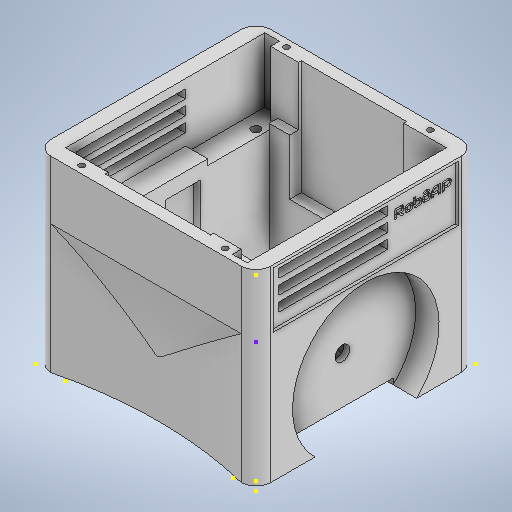
# Autodesk Inventor part: Chassi_VSSS
Saved by Autodesk Inventor 2025.2 (Build 292293000, 293)
## iProperties
Created: 2025-03-20
Part Number: Chassi_VSSS
Material: Genérico
Document SubType Name: Modeling
Designer: miche
Density: 1 g/cm^3
Appearance: Padrão
Author: miche
Autodesk Inventor part; units mm, degrees
(part 1 of 2)
ref_plane "YZ Plane" through (0, 0, 0) normal (1, 0, 0) x (0, 1, 0)
ref_plane "XZ Plane" through (0, 0, 0) normal (0, 1, 0) x (-1, 0, 0)
ref_plane "XY Plane" through (0, 0, 0) normal (0, 0, 1) x (1, 0, 0)
sketch "Esboço1" plane through (0, 0, 0) normal (0, 1, 0) x (-1, 0, 0)
  line L0 (5, 0) -> (70, 0)
  line L1 (75, -5) -> (75, -70)
  line L2 (70, -75) -> (5, -75)
  line L3 (0, -70) -> (0, -5)
  arc A0 (75, -5) -> (70, 0) centre (70, -5) ccw
  arc A1 (70, -75) -> (75, -70) centre (70, -70) ccw
  arc A2 (0, -70) -> (5, -75) centre (5, -70) ccw
  arc A3 (5, 0) -> (0, -5) centre (5, -5) ccw
  point P0 (0, 0)
  point P1 (75, -75)
  point P2 (75, 0)
  point P3 (0, -75)
  dimension "d0" = 75
  dimension "d1" = 75
  dimension "d2" = 5
  dimension "d3" = 5
  constraints: 8 end point, 8 point on circle, 8 point on line, 8 tangent, 4 centre point, 2 equal radius, 2 parallel, 1 horizontal, 1 perpendicular
  measures "d0" distance of point (75, -75) point (0, -75)
  measures "d1" distance of point (75, 0) point (75, -75)
  measures "d2" radius of A0
  measures "d3" radius of A3
extrude "Extrusão1" add sketch "Esboço1" along normal blind 3
sketch "Esboço2" plane through (0, 3, 0) normal (0, 1, 0) x (1, 0, 0)
  arc A0 (-70, 75) -> (-75, 70) centre (-70, 70) ccw projected
  line L0 (-70, 75) -> (-70, 70)
  line L1 (-70, 70) -> (-75, 70)
  line L2 (-70, 70) -> (-70, 5)
  line L3 (-70, 5) -> (-75, 5)
  line L4 (-75, 5) -> (-75, 70)
  line L5 (-70, 70) -> (-5, 70)
  line L6 (-5, 70) -> (-5, 5)
  line L7 (-5, 5) -> (-70, 5)
  line L8 (-5, 70) -> (0, 70)
  line L9 (0, 70) -> (0, 5)
  line L10 (0, 5) -> (-5, 5)
  line L11 (-5, 5) -> (-5, 0)
  line L12 (-5, 0) -> (-70, 0)
  line L13 (-70, 0) -> (-70, 5)
  line L14 (-5, 75) -> (-70, 75) projected
  line L15 (-5, 75) -> (-5, 70)
  arc A1 (-70, 75) -> (-75, 70) centre (-70, 70) ccw
  arc A2 (0, 70) -> (-5, 75) centre (-5, 70) ccw projected
  arc A3 (0, 70) -> (-5, 75) centre (-5, 70) ccw
  arc A4 (-5, 0) -> (0, 5) centre (-5, 5) ccw projected
  arc A5 (-5, 0) -> (0, 5) centre (-5, 5) ccw
  arc A6 (-75, 5) -> (-70, 0) centre (-70, 5) ccw
  line L16 (-70, 70) -> (-65, 70)
  line L17 (-65, 70) -> (-65, 5)
  line L18 (-65, 5) -> (-70, 5)
  line L19 (-70, 5) -> (-70, 70)
  line L20 (-5, 70) -> (-10, 70)
  line L21 (-10, 70) -> (-10, 5)
  line L22 (-10, 5) -> (-5, 5)
  line L23 (-5, 5) -> (-5, 70)
  line L24 (-70, 70) -> (-70, 71)
  line L25 (-70, 70) -> (-5, 70)
  line L26 (-5, 70) -> (-5, 71)
  line L27 (-5, 71) -> (-70, 71)
  line L28 (-70, 71) -> (-70, 70)
  line L29 (-70, 5) -> (-5, 5)
  line L30 (-5, 5) -> (-5, 4)
  line L31 (-5, 4) -> (-70, 4)
  line L32 (-70, 4) -> (-70, 5)
  arc A7 (-70, 75) -> (-5, 75) centre (-37.5, 205.0313) ccw
  arc A8 (-5, 0) -> (-70, 0) centre (-37.5, -130.0312) ccw
  point P0 (0, 0)
  constraints: 64 end point, 13 perpendicular, 13 point on circle, 10 point on line, 9 parallel, 6 centre point, 5 horizontal, 2 tangent, 2 vertical
extrude "Extrusão2" add sketch "Esboço2" along normal blind 15 contours L1 L2 L3 L4 | L5 L17 L7 L2 | L9 L10 L6 L8 | L6 L7 L21 L5
extrude "Extrusão3" cut sketch "Esboço2" against normal blind 3 contours L14 A7 | A8 L12
extrude "Extrusão4" add sketch "Esboço2" along normal blind 15 contours L0 L1 A0 | A7 L27 L0 | L27 L15 L5 L0 | A2 L8 L15 | L15 L27 A7 | L3 L13 A6 | L7 L11 L31 L13 | L13 L31 A8 | A4 L11 L10 | A8 L31 L11
sketch "Esboço3" plane through (-75, 0, -70) normal (-1, 0, 0) x (0, 0, 1)
  line L0 (65, 18) -> (0, 18) projected
  line L1 (32.5, 18) -> (32.5, 0)
  circle A0 centre (32.5, 18) radius 25
  circle A1 centre (32.5, 18) radius 2.5
  point P0 (70, 0)
  dimension "d35" = 5
  constraints: 2 centre point, 2 coincident, 2 end point, 1 midpoint, 1 vertical
  measures "d35" diameter of A1
sketch "Esboço4" plane through (0, 0, -5) normal (1, 0, 0) x (0, 0, -1)
  line L0 (0, 18) -> (65, 18) projected
  line L1 (32.5, 18) -> (32.5, 0)
  line L2 (0, 0) -> (65, 0) projected
  circle A0 centre (32.5, 18) radius 25
  circle A1 centre (32.5, 18) radius 2.5
  point P0 (-5, 0)
  dimension "d12" = 50
  dimension "d30" = 5
  constraints: 2 centre point, 2 coincident, 2 end point, 2 midpoint
  measures "d12" diameter of A0
  measures "d30" diameter of A1
sketch "Esboço5" plane through (0, 18, 0) normal (0, 1, 0) x (1, 0, 0)
  line L0 (-10, 70) -> (-10, 5) projected
  line L1 (-10, 5) -> (0, 5)
  line L2 (0, 5) -> (0, 70)
  line L3 (0, 70) -> (-10, 70)
  line L4 (-10, 70) -> (-10, 5)
  line L5 (-75, 70) -> (-75, 5) projected
  line L6 (-65, 70) -> (-65, 5) projected
  line L7 (-75, 5) -> (-65, 5)
  line L8 (-65, 5) -> (-65, 70)
  line L9 (-65, 70) -> (-75, 70)
  line L10 (-75, 70) -> (-75, 5)
  point P0 (0, 0)
  constraints: 16 end point, 4 parallel, 2 horizontal, 2 perpendicular
extrude "Extrusão5" add sketch "Esboço5" along normal blind 26
sketch "Esboço6" plane through (0, 18, 0) normal (0, 1, 0) x (1, 0, 0)
  arc A0 (0, 70) -> (-5, 75) centre (-5, 70) ccw projected
  line L0 (-5, 75) -> (-5, 70)
  line L1 (-5, 70) -> (0, 70)
  point P0 (0, 0)
  constraints: 4 end point, 1 perpendicular, 1 vertical
extrude "Extrusão6" add sketch "Esboço6" along normal blind 26
sketch "Esboço7" plane through (-5, 18, -75) normal (-1, 0, 0) x (0, 0, 1)
  line L0 (5, 26) -> (0, 26) projected
  line L1 (5, 26) -> (4, 26)
  line L2 (4, 26) -> (4, 0)
  line L3 (4, 0) -> (5, 0)
  line L4 (5, 0) -> (5, 26)
  arc A0 (4, 0) -> (0, 26) centre (-79.25, 0.5) ccw
  line L5 (0, 26) -> (4, 26)
  point P0 (75, -18)
  point P1 (4, 1)
  point P2 (4, 26)
  constraints: 10 end point, 2 parallel, 2 point on circle, 1 centre point, 1 collinear, 1 horizontal, 1 perpendicular
sketch "Esboço8" plane through (0, 18, 0) normal (0, 1, 0) x (1, 0, 0)
  line L0 (-5, 70) -> (-10, 70) projected
  arc A0 (-70, 75) -> (-5, 75) centre (-37.5, 205.0313) ccw projected
  line L1 (-5, 70) -> (-5, 75)
  line L2 (-75, 70) -> (-65, 70) projected
  line L3 (-5, 70) -> (-75, 70)
  arc A1 (-70, 75) -> (-75, 70) centre (-70, 70) ccw projected
  arc A2 (-70, 75) -> (-75, 70) centre (-70, 70) ccw
  arc A3 (-70, 75) -> (-5, 75) centre (-37.5, 205.0313) ccw
  point P0 (0, 0)
  constraints: 4 end point, 4 point on circle, 2 centre point, 1 collinear, 1 concentric, 1 vertical
extrude "Extrusão7" add sketch "Esboço8" along normal blind 26
extrude "Extrusão8" add sketch "Esboço7" along normal blind 65
sketch "Esboço9" plane through (0, 18, 0) normal (0, 1, 0) x (1, 0, 0)
  arc A0 (-5, 0) -> (-70, 0) centre (-37.5, -130.0312) ccw projected
  line L0 (-70, 0) -> (-70, 5)
  line L1 (-65, 5) -> (-75, 5) projected
  line L2 (-70, 5) -> (-75, 5)
  arc A1 (-75, 5) -> (-70, 0) centre (-70, 5) ccw projected
  arc A2 (-75, 5) -> (-70, 0) centre (-70, 5) ccw
  line L3 (-70, 5) -> (0, 5)
  arc A3 (-5, 0) -> (-70, 0) centre (-37.5, -130.0312) ccw
  arc A4 (-5, 0) -> (0, 5) centre (-5, 5) ccw projected
  arc A5 (-5, 0) -> (0, 5) centre (-5, 5) ccw
  point P0 (0, 0)
  constraints: 6 end point, 6 point on circle, 3 centre point, 1 collinear, 1 concentric, 1 point on line, 1 vertical
extrude "Extrusão9" add sketch "Esboço9" along normal blind 26 contours A1 L1 L0
sketch "Esboço13" plane through (0, 18, 0) normal (0, 1, 0) x (1, 0, 0)
  line L0 (-70, 5) -> (-70, 0) projected
  line L1 (-10, 5) -> (0, 5) projected
  line L2 (-70, 5) -> (0, 5)
  arc A0 (-5, 0) -> (-70, 0) centre (-37.5, -130.0312) ccw projected
  line L3 (-5, 0) -> (-5, 4)
  line L4 (-70, 0) -> (-70, 4)
  line L5 (-70, 4) -> (-5, 4)
  arc A1 (-5, 0) -> (-70, 0) centre (-37.5, -130.0312) ccw
  arc A2 (-5, 0) -> (0, 5) centre (-5, 5) ccw projected
  arc A3 (-5, 0) -> (0, 5) centre (-5, 5) ccw
  point P0 (0, 0)
  constraints: 8 end point, 4 point on circle, 2 centre point, 1 collinear, 1 parallel, 1 point on line, 1 vertical
sketch "Esboço14" plane through (-70, 18, 0) normal (1, 0, 0) x (0, 0, -1)
  line L0 (5, 26) -> (0, 26) projected
  line L1 (5, 26) -> (4, 26)
  line L2 (4, 0) -> (4, -18) projected
  line L3 (4, 0) -> (4, 26)
  line L4 (0, 26) -> (4, 26)
  arc A0 (4, 0) -> (0, 26) centre (-79.25, 0.5) ccw
  point P0 (0, -18)
  point P1 (0, 26)
  point P2 (4, 1)
  constraints: 6 end point, 3 point on line, 2 point on circle, 1 centre point, 1 collinear, 1 perpendicular
extrude "Extrusão11" add sketch "Esboço13" along normal blind 26
extrude "Extrusão12" add sketch "Esboço14" along normal blind 65
extrude "Extrusão13" cut sketch "Esboço4" against normal blind 8 contours A1 L0 A0 | L0 A0 L2 L1 A1 | A1 L1 L2 A0 L0 | L2 A0
sketch "Esboço15" plane through (0, 18, -37.5) normal (1, 0, 0) x (0, 0, -1)
  circle A0 centre (0, 0) radius 2.5 projected
  circle A1 centre (0, 0) radius 2.5
  point P0 (-37.5, -18)
  constraints: 1 centre point, 1 coincident
extrude "Extrusão14" cut sketch "Esboço15" against normal blind 10
sketch "Esboço16" plane through (-75, 0, -70) normal (-1, 0, 0) x (0, 0, 1)
  point P0 (70, 0)
extrude "Extrusão15" cut sketch "Esboço3" against normal blind 8 contours A0 L0 A1 | L0 A1 A0
extrude "Extrusão16" cut sketch "Esboço3" against normal blind 10 contours A1 L1 L0 | L0 A1 | L1 A1 L0
sketch "Esboço17" plane through (0, 3, 0) normal (0, 1, 0) x (1, 0, 0)
  point P0 (0, 0)
sketch "Esboço18" plane through (-65, 3, -5) normal (1, 0, 0) x (0, 0, -1)
  circle A0 centre (32.5, 15) radius 2.5 projected
  line L0 (32.5, 15) -> (32.5, 13)
  line L1 (32.5, 13) -> (32.5, 9)
  line L2 (32.5, 9) -> (38.5, 9)
  line L3 (32.5, 9) -> (26.5, 9)
  line L4 (32.5, 9) -> (38.5, 9) construction
  line L5 (26.5, 9) -> (26.5, 0)
  line L6 (65, 0) -> (0, 0) projected
  line L7 (38.5, 9) -> (38.5, 0)
  line L8 (15.1506, -3) -> (49.8494, -3) projected
  line L9 (38.5, 9) -> (47.5, 9) construction
  line L10 (26.5, 0) -> (38.5, 0)
  point P0 (-5, -3)
  point P1 (38.5, 0)
  point P2 (38.5, 9)
  dimension "d40" = 2
  dimension "d44" = 6
  dimension "d45" = 6
  dimension "d46" = 180
  dimension "d47" = 9
  dimension "d48" = 90
  constraints: 18 end point, 4 horizontal, 3 vertical, 2 equal length, 2 perpendicular, 1 point on line
  measures "d40" distance of L0.start L0.end
  measures "d44" distance of L1.end L2.end
  measures "d45" distance of L1.end L3.end
  measures "d46" angle of L3 L4
  measures "d47" distance of L4.end L7.end
  measures "d48" angle of L7 L9
extrude "Extrusão17" add sketch "Esboço18" along normal blind 55 contours L2 L7 L6 L5 L3
sketch "Esboço19" plane through (0, 3, 0) normal (0, 1, 0) x (1, 0, 0)
  line L0 (-65, 31.5) -> (-10, 31.5) projected
  line L1 (-65, 31.5) -> (-65, 5) projected
  line L2 (-10, 31.5) -> (-65, 31.5)
  line L3 (-65, 31.5) -> (-65, 26.5)
  line L4 (-65, 26.5) -> (-10, 26.5)
  line L5 (-10, 26.5) -> (-10, 31.5)
  line L6 (-10, 43.5) -> (-10, 31.5) projected
  line L7 (-10, 43.5) -> (-65, 43.5)
  line L8 (-65, 43.5) -> (-65, 48.5)
  line L9 (-65, 48.5) -> (-10, 48.5)
  line L10 (-10, 48.5) -> (-10, 43.5)
  point P0 (0, 0)
  dimension "d51" = 5
  dimension "d52" = 5
  constraints: 16 end point, 4 parallel, 2 horizontal, 2 perpendicular, 1 point on line
  measures "d51" distance of L3.end L2.end
  measures "d52" distance of L7.end L8.end
extrude "Extrusão18" add sketch "Esboço19" along normal blind 13
sketch "Esboço20" plane through (-8, 0, -5) normal (1, 0, 0) x (0, 0, -1)
  point P0 (-5, 0)
sketch "Esboço21" plane through (0, 3, 0) normal (0, 1, 0) x (1, 0, 0)
  line L0 (-10, 48.5) -> (-65, 48.5) projected
  line L1 (-10, 48.5) -> (-10, 70) projected
  line L2 (-65, 48.5) -> (-10, 48.5)
  line L3 (-10, 48.5) -> (-10, 51.5)
  line L4 (-10, 51.5) -> (-65, 51.5)
  line L5 (-65, 51.5) -> (-65, 48.5)
  line L6 (-65, 26.5) -> (-10, 26.5) projected
  line L7 (-65, 26.5) -> (-10, 26.5)
  line L8 (-10, 26.5) -> (-10, 23.5)
  line L9 (-10, 23.5) -> (-65, 23.5)
  line L10 (-65, 23.5) -> (-65, 26.5)
  point P0 (0, 0)
  dimension "d55" = 3
  dimension "d56" = 55
  dimension "d57" = 3
  constraints: 16 end point, 4 parallel, 2 horizontal, 2 perpendicular, 1 point on line
  measures "d55" distance of L3.end L2.end
  measures "d56" distance of L8.end L9.end
  measures "d57" distance of L7.end L8.end
extrude "Extrusão19" add sketch "Esboço21" along normal blind 13
sketch "Esboço22" plane through (0, 3, 0) normal (0, 1, 0) x (1, 0, 0)
  line L0 (-65, 5) -> (-65, 70) projected
  line L1 (-10, 70) -> (-10, 5) projected
  line L2 (-65, 70) -> (-10, 70)
  line L3 (-10, 70) -> (-10, 67)
  line L4 (-10, 67) -> (-65, 67)
  line L5 (-65, 67) -> (-65, 70)
  line L6 (-65, 5) -> (-10, 5)
  line L7 (-10, 5) -> (-10, 8)
  line L8 (-10, 8) -> (-65, 8)
  line L9 (-65, 8) -> (-65, 5)
  point P0 (0, 0)
  constraints: 16 end point, 4 parallel, 2 horizontal, 2 perpendicular, 2 point on line
extrude "Extrusão20" add sketch "Esboço22" along normal blind 41 contours L0 L8 L1 L6 | L0 L2 L1 L4
sketch "Esboço23" plane through (0, 16, 0) normal (0, 1, 0) x (1, 0, 0)
  line L0 (-65, 43.5) -> (-10, 43.5) projected
  line L1 (-65, 43.5) -> (-41, 43.5)
  line L2 (-10, 43.5) -> (-34, 43.5)
  line L3 (-34, 43.5) -> (-34, 31.5)
  line L4 (-10, 31.5) -> (-65, 31.5) projected
  line L5 (-41, 43.5) -> (-41, 31.5)
  line L6 (-41, 43.5) -> (-41, 51.5)
  line L7 (-10, 51.5) -> (-65, 51.5) projected
  line L8 (-34, 31.5) -> (-34, 23.5)
  line L9 (-10, 23.5) -> (-65, 23.5) projected
  point P0 (0, 0)
  dimension "d62" = 24
  constraints: 12 end point, 5 point on line, 3 vertical, 1 perpendicular
  measures "d62" distance of L0.start L1.end
sketch "Esboço24" plane through (0, 16, 0) normal (0, 1, 0) x (1, 0, 0)
  line L0 (-10, 51.5) -> (-65, 51.5) projected
  line L1 (-10, 23.5) -> (-65, 23.5) projected
  line L2 (-41, 51.5) -> (-34, 51.5)
  line L3 (-34, 51.5) -> (-34, 23.5)
  line L4 (-34, 23.5) -> (-41, 23.5)
  line L5 (-41, 23.5) -> (-41, 51.5)
  point P0 (0, 0)
  constraints: 8 end point, 2 parallel, 2 point on line, 1 horizontal, 1 perpendicular
extrude "Extrusão21" cut sketch "Esboço24" against normal blind 13
sketch "Esboço25" plane through (0, 3, 0) normal (0, 1, 0) x (1, 0, 0)
  line L0 (-10, 51.5) -> (-34, 51.5) projected
  line L1 (-65, 67) -> (-10, 67)
  line L2 (-10, 67) -> (-10, 51.5)
  line L3 (-10, 51.5) -> (-65, 51.5)
  line L4 (-65, 51.5) -> (-65, 67)
  line L5 (-65, 23.5) -> (-65, 8) projected
  line L6 (-10, 23.5) -> (-34, 23.5) projected
  line L7 (-65, 8) -> (-10, 8)
  line L8 (-10, 8) -> (-10, 23.5)
  line L9 (-10, 23.5) -> (-65, 23.5)
  line L10 (-65, 23.5) -> (-65, 8)
  point P0 (0, 0)
  constraints: 16 end point, 4 parallel, 2 horizontal, 2 perpendicular
extrude "Extrusão22" cut sketch "Esboço25" against normal blind 3
sketch "Esboço26" plane through (0, 3, 0) normal (0, 1, 0) x (1, 0, 0)
  point P0 (0, 0)
sketch "Esboço27" plane through (0, 3, 0) normal (0, 1, 0) x (1, 0, 0)
  line L0 (-41, 51.5) -> (-65, 51.5) projected
  line L1 (-34, 51.5) -> (-34, 43.5) projected
  line L2 (-41, 51.5) -> (-34, 51.5)
  line L3 (-34, 51.5) -> (-34, 43.5)
  line L4 (-34, 43.5) -> (-41, 43.5)
  line L5 (-41, 43.5) -> (-41, 51.5)
  line L6 (-41, 23.5) -> (-34, 23.5) projected
  line L7 (-41, 23.5) -> (-41, 31.5) projected
  line L8 (-34, 23.5) -> (-41, 23.5)
  line L9 (-41, 23.5) -> (-41, 31.5)
  line L10 (-41, 31.5) -> (-34, 31.5)
  line L11 (-34, 31.5) -> (-34, 23.5)
  point P0 (0, 0)
  constraints: 16 end point, 4 parallel, 2 horizontal, 2 perpendicular
extrude "Extrusão23" cut sketch "Esboço27" against normal blind 3
sketch "Esboço28" plane through (0, 16, 0) normal (0, 1, 0) x (1, 0, 0)
  line L0 (-65, 43.5) -> (-53, 43.5)
  line L1 (-65, 43.5) -> (-41, 43.5) projected
  line L2 (-41, 31.5) -> (-65, 31.5) projected
  line L3 (-65, 31.5) -> (-53, 31.5)
  line L4 (-10, 43.5) -> (-10, 31.5) projected
  line L5 (-10, 43.5) -> (-22, 43.5)
  line L6 (-10, 31.5) -> (-22, 31.5)
  line L7 (-53, 43.5) -> (-53, 47.5)
  line L8 (-53, 31.5) -> (-53, 27.5)
  line L9 (-22, 43.5) -> (-22, 47.5)
  line L10 (-34, 43.5) -> (-10, 43.5) projected
  line L11 (-22, 43.5) -> (-18, 43.5) construction
  line L12 (-22, 31.5) -> (-22, 27.5)
  circle A0 centre (-53, 47.5) radius 1.5
  circle A1 centre (-22, 47.5) radius 1.5
  circle A2 centre (-53, 27.5) radius 1.5
  circle A3 centre (-22, 27.5) radius 1.5
  point P0 (0, 0)
  dimension "d69" = 4
  dimension "d70" = 4
  dimension "d71" = 4
  dimension "d72" = 90
  dimension "d73" = 3
  dimension "d74" = 3
  dimension "d75" = 3
  dimension "d76" = 3
  constraints: 18 end point, 4 centre point, 4 coincident, 3 perpendicular, 2 midpoint, 2 point on line, 2 vertical, 1 horizontal
  measures "d69" distance of L0.end L7.end
  measures "d70" distance of L3.end L8.end
  measures "d71" distance of L5.end L9.end
  measures "d72" angle of L11 L9
  measures "d73" diameter of A0
  measures "d74" diameter of A1
  measures "d75" diameter of A2
  measures "d76" diameter of A3
extrude "Extrusão24" cut sketch "Esboço28" against normal blind 10
thread "Rosca1" size "M3x0.5" class "6H" standard "ANSI Metric M Profile" full length
thread "Rosca2" size "M3x0.5" class "6H" standard "ANSI Metric M Profile" full length
thread "Rosca3" size "M3x0.5" class "6H" standard "ANSI Metric M Profile" full length
thread "Rosca4" size "M3x0.5" class "6H" standard "ANSI Metric M Profile" full length
sketch "Esboço29" plane through (0, 3, 0) normal (0, 1, 0) x (1, 0, 0)
  line L0 (-41, 31.5) -> (-41, 23.5) projected
  line L1 (-34, 43.5) -> (-34, 31.5) projected
  line L2 (-41, 31.5) -> (-34, 31.5)
  line L3 (-34, 31.5) -> (-34, 43.5)
  line L4 (-34, 43.5) -> (-41, 43.5)
  line L5 (-41, 43.5) -> (-41, 31.5)
  point P0 (0, 0)
  constraints: 8 end point, 2 parallel, 1 horizontal, 1 perpendicular
extrude "Extrusão25" add sketch "Esboço29" along normal blind 13
sketch "Esboço30" plane through (0, 44, 0) normal (0, 1, 0) x (1, 0, 0)
  point P0 (0, 0)
sketch "Esboço31" plane through (0, 44, 0) normal (0, 1, 0) x (1, 0, 0)
  line L0 (-5, 75) -> (-70, 75) projected
  arc A0 (-70, 75) -> (-75, 70) centre (-70, 70) ccw projected
  line L1 (-70, 75) -> (-70, 70)
  line L2 (-70, 70) -> (-5, 70)
  line L3 (-5, 70) -> (-5, 75)
  line L4 (-70, 70) -> (-70, 5)
  line L5 (-70, 5) -> (-5, 5)
  line L6 (-5, 5) -> (-5, 70)
  line L7 (-75, 70) -> (-75, 5) projected
  line L8 (-75, 70) -> (-75, 5)
  arc A1 (-75, 5) -> (-70, 0) centre (-70, 5) ccw projected
  arc A2 (-5, 0) -> (-70, 0) centre (-37.5, -130.0312) ccw projected
  line L9 (-70, 0) -> (-5, 0)
  line L10 (0, 5) -> (0, 20.1506) projected
  line L11 (0, 70) -> (0, 5)
  line L12 (-70, 75) -> (-5, 75)
  arc A3 (-70, 75) -> (-75, 70) centre (-70, 70) ccw
  arc A4 (0, 70) -> (-5, 75) centre (-5, 70) ccw
  arc A5 (-75, 5) -> (-70, 0) centre (-70, 5) ccw
  arc A6 (-5, 0) -> (0, 5) centre (-5, 5) ccw
  point P0 (0, 0)
  dimension "d89" = 65
  dimension "d90" = 65
  constraints: 20 end point, 8 point on circle, 4 centre point, 4 perpendicular, 3 vertical, 2 collinear, 2 tangent, 1 concentric, 1 horizontal
  measures "d89" distance of L1.end L4.end
  measures "d90" distance of L4.end L5.end
extrude "Extrusão26" add sketch "Esboço31" along normal blind 20 contours L3 L2 L1 L0 | A4 L11 L10 A6 A2 A1 L7 A0 L1 L4 L5 L6 L3 | A2 L9
sketch "Esboço32" plane through (-65, 12, -31.5) normal (1, 0, 0) x (0, 0, -1)
  line L0 (20, 4) -> (20, -12) projected
  point P0 (-31.5, -12)
sketch "Esboço33" plane through (0, 44, 0) normal (0, 1, 0) x (1, 0, 0)
  line L0 (-65, 67) -> (-55.5, 67)
  line L1 (-65, 67) -> (-10, 67) projected
  line L2 (-55.5, 67) -> (-55.5, 70)
  line L3 (-55.5, 67) -> (-19.5, 67)
  line L4 (-19.5, 67) -> (-10, 67)
  line L5 (-19.5, 67) -> (-19.5, 70)
  line L6 (-55.5, 70) -> (-19.5, 70)
  line L7 (-5, 70) -> (-70, 70) projected
  line L8 (-55.5, 67) -> (-55.5, 8)
  line L9 (-10, 8) -> (-65, 8) projected
  line L10 (-55.5, 67) -> (3.5, 67) construction
  line L11 (-55.5, 8) -> (-19.5, 8)
  line L12 (-55.5, 8) -> (-55.5, 5)
  line L13 (-70, 5) -> (-5, 5) projected
  line L14 (-19.5, 8) -> (-19.5, 5)
  line L15 (-55.5, 5) -> (-19.5, 5)
  point P0 (0, 0)
  dimension "d93" = 9.5
  dimension "d94" = 36
  dimension "d95" = 59
  dimension "d96" = 90
  dimension "d97" = 36
  constraints: 24 end point, 5 point on line, 3 collinear, 3 perpendicular, 2 vertical, 1 horizontal, 1 parallel
  measures "d93" distance of L0.start L0.end
  measures "d94" distance of L0.end L3.end
  measures "d95" distance of L0.end L8.end
  measures "d96" angle of L8 L10
  measures "d97" distance of L8.end L11.end
extrude "Extrusão27" cut sketch "Esboço33" against normal blind 19
sketch "Esboço34" plane through (0, 64, 0) normal (0, 1, 0) x (1, 0, 0)
  point P0 (0, 0)
sketch "Esboço35" plane through (0, 64, 0) normal (0, 1, 0) x (1, 0, 0)
  line L0 (-19.5, 70) -> (-19.5, 67) projected
  line L1 (-19.5, 70) -> (-55.5, 70)
  line L2 (-55.5, 70) -> (-55.5, 71)
  line L3 (-55.5, 71) -> (-19.5, 71)
  line L4 (-19.5, 71) -> (-19.5, 70)
  line L5 (-19.5, 5) -> (-55.5, 5)
  line L6 (-55.5, 5) -> (-55.5, 4)
  line L7 (-55.5, 4) -> (-19.5, 4)
  line L8 (-19.5, 4) -> (-19.5, 5)
  point P0 (0, 0)
  constraints: 16 end point, 4 parallel, 2 horizontal, 2 perpendicular
extrude "Extrusão28" cut sketch "Esboço35" against normal blind 39
sketch "Esboço36" plane through (0, 0, -54.8494) normal (1, 0, 0) x (0, 0, -1)
  point P0 (-54.8494, 0)
sketch "Esboço37" plane through (0, 0, -54.8494) normal (1, 0, 0) x (0, 0, -1)
  line L0 (-38.5511, 65.9897) -> (44.7833, 65.9897) construction
  line L1 (44.7833, 65.9897) -> (44.7833, 48.6358) construction
  line L2 (44.7833, 48.6358) -> (-38.5511, 48.6358) construction
  line L3 (-38.5511, 48.6358) -> (-38.5511, 65.9897) construction
  spline S0 degree 2 poles (-3.3485, 57.5742) (-3.3485, 57.3818) (-3.4433, 57.0784) (-3.6086, 56.8426) (-3.8199, 56.6774) (-4.0529, 56.5717) (-4.2887, 56.5229) (-4.3483, 56.5229) knots 0 0 0 1 2 3 4 5 6 6 6
  line L4 (-4.3483, 56.5229) -> (-3.2184, 55.5475)
  line L5 (-3.2184, 55.5475) -> (-4.118, 55.5475)
  line L6 (-4.118, 55.5475) -> (-5.2478, 56.5229)
  line L7 (-5.2478, 56.5229) -> (-5.6623, 56.5229)
  line L8 (-5.6623, 56.5229) -> (-5.6623, 57.1515)
  line L9 (-5.6623, 57.1515) -> (-4.3916, 57.1515)
  spline S1 degree 2 poles (-4.3916, 57.1515) (-4.3049, 57.1596) (-4.1478, 57.222) (-4.0394, 57.3276) (-3.9771, 57.4766) (-3.9771, 57.5742) knots 0 0 0 1 2 3 4 4 4
  line L10 (-3.9771, 57.5742) -> (-3.9771, 57.9156)
  spline S2 degree 2 poles (-3.9771, 57.9156) (-3.9771, 57.9508) (-3.9906, 57.9779) (-4.0069, 57.9887) (-4.0367, 57.9914) (-4.0502, 57.9914) knots 0 0 0 1 2 3 4 4 4
  line L11 (-4.0502, 57.9914) -> (-5.7897, 57.9914)
  line L12 (-5.7897, 57.9914) -> (-5.7897, 55.5475)
  line L13 (-5.7897, 55.5475) -> (-6.421, 55.5475)
  line L14 (-6.421, 55.5475) -> (-6.421, 58.303)
  spline S3 degree 2 poles (-6.421, 58.303) (-6.421, 58.3707) (-6.3749, 58.4845) (-6.2882, 58.5712) (-6.1717, 58.62) (-6.104, 58.62) knots 0 0 0 1 2 3 4 4 4
  line L15 (-6.104, 58.62) -> (-4.0502, 58.62)
  spline S4 degree 2 poles (-4.0502, 58.62) (-3.8579, 58.62) (-3.5869, 58.4791) (-3.4216, 58.2678) (-3.3485, 58.0239) (-3.3485, 57.9183) knots 0 0 0 1 2 3 4 4 4
  line L16 (-3.3485, 57.9183) -> (-3.3485, 57.5742)
  spline S5 degree 2 poles (-0.3383, 56.3522) (-0.3383, 56.2059) (-0.4142, 55.9702) (-0.5388, 55.7914) (-0.7014, 55.664) (-0.8802, 55.5855) (-1.0645, 55.5475) (-1.1457, 55.5475) knots 0 0 0 1 2 3 4 5 6 6 6
  line L17 (-1.1457, 55.5475) -> (-2.1211, 55.5475)
  spline S6 degree 2 poles (-2.1211, 55.5475) (-2.2431, 55.5475) (-2.5221, 55.6315) (-2.7633, 55.8212) (-2.9231, 56.1301) (-2.9231, 56.3522) knots 0 0 0 1 2 3 4 4 4
  line L18 (-2.9231, 56.3522) -> (-2.9231, 57.0838)
  spline S7 degree 2 poles (-2.9231, 57.0838) (-2.9231, 57.3032) (-2.7633, 57.6094) (-2.5221, 57.8018) (-2.2403, 57.8858) (-2.1211, 57.8858) knots 0 0 0 1 2 3 4 4 4
  line L19 (-2.1211, 57.8858) -> (-1.1457, 57.8858)
  spline S8 degree 2 poles (-1.1457, 57.8858) (-0.9263, 57.8858) (-0.6147, 57.7259) (-0.425, 57.4848) (-0.3383, 57.203) (-0.3383, 57.0838) knots 0 0 0 1 2 3 4 4 4
  line L20 (-0.3383, 57.0838) -> (-0.3383, 56.3522)
  spline S9 degree 2 poles (-0.9696, 57.0811) (-0.9696, 57.1732) (-1.059, 57.2572) (-1.1457, 57.2572) knots 0 0 0 1 2 2 2
  line L21 (-1.1457, 57.2572) -> (-2.1184, 57.2572)
  spline S10 degree 2 poles (-2.1184, 57.2572) (-2.2078, 57.2572) (-2.2918, 57.1732) (-2.2918, 57.0838) knots 0 0 0 1 2 2 2
  line L22 (-2.2918, 57.0838) -> (-2.2918, 56.3522)
  spline S11 degree 2 poles (-2.2918, 56.3522) (-2.2918, 56.2628) (-2.2078, 56.1761) (-2.1184, 56.1761) knots 0 0 0 1 2 2 2
  line L23 (-2.1184, 56.1761) -> (-1.1457, 56.1761)
  spline S12 degree 2 poles (-1.1457, 56.1761) (-1.0536, 56.1761) (-0.9696, 56.2628) (-0.9696, 56.3522) knots 0 0 0 1 2 2 2
  line L24 (-0.9696, 56.3522) -> (-0.9696, 57.0811)
  spline S13 degree 2 poles (2.6664, 56.3522) (2.6664, 56.271) (2.6285, 56.0894) (2.5499, 55.9133) (2.4252, 55.7507) (2.2437, 55.6234) (2.008, 55.5475) (1.8617, 55.5475) knots 0 0 0 1 2 3 4 5 6 6 6
  line L25 (1.8617, 55.5475) -> (0.8863, 55.5475)
  spline S14 degree 2 poles (0.8863, 55.5475) (0.8023, 55.5475) (0.6235, 55.5855) (0.4447, 55.664) (0.2821, 55.7887) (0.1575, 55.9675) (0.0816, 56.2032) (0.0816, 56.3522) knots 0 0 0 1 2 3 4 5 6 6 6
  line L26 (0.0816, 56.3522) -> (0.0816, 58.8368)
  line L27 (0.0816, 58.8368) -> (0.7129, 58.8368)
  line L28 (0.7129, 58.8368) -> (0.7129, 56.3522)
  spline S15 degree 2 poles (0.7129, 56.3522) (0.7129, 56.2682) (0.8104, 56.1761) (0.8863, 56.1761) knots 0 0 0 1 2 2 2
  line L29 (0.8863, 56.1761) -> (1.8617, 56.1761)
  spline S16 degree 2 poles (1.8617, 56.1761) (1.9457, 56.1761) (2.0351, 56.271) (2.0351, 56.3522) knots 0 0 0 1 2 2 2
  line L30 (2.0351, 56.3522) -> (2.0351, 57.0838)
  spline S17 degree 2 poles (2.0351, 57.0838) (2.0351, 57.1651) (1.9403, 57.2572) (1.8617, 57.2572) knots 0 0 0 1 2 2 2
  line L31 (1.8617, 57.2572) -> (0.843, 57.2572)
  line L32 (0.843, 57.2572) -> (0.843, 57.8858)
  line L33 (0.843, 57.8858) -> (1.8617, 57.8858)
  spline S18 degree 2 poles (1.8617, 57.8858) (1.9403, 57.8858) (2.1245, 57.8478) (2.3033, 57.7665) (2.4659, 57.6419) (2.5905, 57.4631) (2.6664, 57.2274) (2.6664, 57.0838) knots 0 0 0 1 2 3 4 5 6 6 6
  line L34 (2.6664, 57.0838) -> (2.6664, 56.3522)
  spline S19 degree 2 poles (5.6413, 56.3522) (5.6413, 56.2059) (5.5654, 55.9702) (5.4408, 55.7914) (5.2782, 55.664) (5.0994, 55.5855) (4.9152, 55.5475) (4.8339, 55.5475) knots 0 0 0 1 2 3 4 5 6 6 6
  line L35 (4.8339, 55.5475) -> (3.8585, 55.5475)
  spline S20 degree 2 poles (3.8585, 55.5475) (3.7366, 55.5475) (3.4575, 55.6315) (3.2164, 55.8212) (3.0565, 56.1301) (3.0565, 56.3522) knots 0 0 0 1 2 3 4 4 4
  line L36 (3.0565, 56.3522) -> (3.0565, 57.0838)
  spline S21 degree 2 poles (3.0565, 57.0838) (3.0565, 57.3032) (3.2164, 57.6094) (3.4575, 57.8018) (3.7393, 57.8858) (3.8585, 57.8858) knots 0 0 0 1 2 3 4 4 4
  line L37 (3.8585, 57.8858) -> (4.8339, 57.8858)
  spline S22 degree 2 poles (4.8339, 57.8858) (5.0534, 57.8858) (5.3649, 57.7259) (5.5546, 57.4848) (5.6413, 57.203) (5.6413, 57.0838) knots 0 0 0 1 2 3 4 4 4
  line L38 (5.6413, 57.0838) -> (5.6413, 56.3522)
  spline S23 degree 2 poles (5.01, 57.0811) (5.01, 57.1732) (4.9206, 57.2572) (4.8339, 57.2572) knots 0 0 0 1 2 2 2
  line L39 (4.8339, 57.2572) -> (3.8612, 57.2572)
  spline S24 degree 2 poles (3.8612, 57.2572) (3.7718, 57.2572) (3.6878, 57.1732) (3.6878, 57.0838) knots 0 0 0 1 2 2 2
  line L40 (3.6878, 57.0838) -> (3.6878, 56.3522)
  spline S25 degree 2 poles (3.6878, 56.3522) (3.6878, 56.2628) (3.7718, 56.1761) (3.8612, 56.1761) knots 0 0 0 1 2 2 2
  line L41 (3.8612, 56.1761) -> (4.8339, 56.1761)
  spline S26 degree 2 poles (4.8339, 56.1761) (4.926, 56.1761) (5.01, 56.2628) (5.01, 56.3522) knots 0 0 0 1 2 2 2
  line L42 (5.01, 56.3522) -> (5.01, 57.0811)
  line L43 (5.0859, 58.089) -> (4.3462, 58.4629)
  line L44 (4.3462, 58.4629) -> (3.6093, 58.089)
  line L45 (3.6093, 58.089) -> (3.3248, 58.4954)
  line L46 (3.3248, 58.4954) -> (4.3462, 59.0779)
  line L47 (4.3462, 59.0779) -> (5.3677, 58.4954)
  line L48 (5.3677, 58.4954) -> (5.0859, 58.089)
  line L49 (9.1527, 55.5475) -> (8.5241, 55.5475)
  line L50 (8.5241, 55.5475) -> (8.5241, 56.2818)
  line L51 (8.5241, 56.2818) -> (6.7088, 56.2818)
  line L52 (6.7088, 56.2818) -> (6.7088, 55.5475)
  line L53 (6.7088, 55.5475) -> (6.0775, 55.5475)
  line L54 (6.0775, 55.5475) -> (6.0775, 57.0838)
  spline S27 degree 2 poles (6.0775, 57.0838) (6.0775, 57.4197) (6.3105, 57.986) (6.7224, 58.3924) (7.2832, 58.62) (7.6138, 58.62) knots 0 0 0 1 2 3 4 4 4
  line L55 (7.6138, 58.62) -> (8.8357, 58.62)
  spline S28 degree 2 poles (8.8357, 58.62) (8.9007, 58.62) (9.0172, 58.5712) (9.1066, 58.4845) (9.1527, 58.368) (9.1527, 58.303) knots 0 0 0 1 2 3 4 4 4
  line L56 (9.1527, 58.303) -> (9.1527, 55.5475)
  line L57 (6.7088, 56.9077) -> (8.5241, 56.9077)
  line L58 (8.5241, 56.9077) -> (8.5241, 57.9914)
  line L59 (8.5241, 57.9914) -> (7.6138, 57.9914)
  spline S29 degree 2 poles (7.6138, 57.9914) (7.5921, 57.9914) (7.4376, 57.9779) (7.2371, 57.921) (7.015, 57.8072) (6.8307, 57.6067) (6.7088, 57.3032) (6.7088, 57.0838) knots 0 0 0 1 2 3 4 5 6 6 6
  line L60 (6.7088, 57.0838) -> (6.7088, 56.9077)
  spline S30 degree 2 poles (12.8348, 57.3276) (12.8348, 57.1353) (12.7399, 56.8318) (12.5747, 56.5988) (12.3633, 56.4335) (12.1303, 56.3278) (11.8919, 56.2818) (11.7889, 56.2818) knots 0 0 0 1 2 3 4 5 6 6 6
  line L61 (11.7889, 56.2818) -> (10.5209, 56.2818)
  line L62 (10.5209, 56.2818) -> (10.5209, 56.9077)
  line L63 (10.5209, 56.9077) -> (11.7916, 56.9077)
  spline S31 degree 2 poles (11.7916, 56.9077) (11.8811, 56.9158) (12.0355, 56.9781) (12.1439, 57.0838) (12.2062, 57.2328) (12.2062, 57.3276) knots 0 0 0 1 2 3 4 4 4
  line L64 (12.2062, 57.3276) -> (12.2062, 57.5688)
  spline S32 degree 2 poles (12.2062, 57.5688) (12.1953, 57.6636) (12.133, 57.8207) (12.0301, 57.9318) (11.8865, 57.9914) (11.7889, 57.9914) knots 0 0 0 1 2 3 4 4 4
  line L65 (11.7889, 57.9914) -> (10.567, 57.9914)
  spline S33 degree 2 poles (10.567, 57.9914) (10.4803, 57.9914) (10.3936, 57.9047) (10.3936, 57.818) knots 0 0 0 1 2 2 2
  line L66 (10.3936, 57.818) -> (10.3936, 55.5475)
  line L67 (10.3936, 55.5475) -> (9.7623, 55.5475)
  line L68 (9.7623, 55.5475) -> (9.7623, 57.818)
  spline S34 degree 2 poles (9.7623, 57.818) (9.7623, 58.0348) (9.9249, 58.3464) (10.1633, 58.536) (10.4451, 58.62) (10.5643, 58.62) knots 0 0 0 1 2 3 4 4 4
  line L69 (10.5643, 58.62) -> (11.7889, 58.62)
  spline S35 degree 2 poles (11.7889, 58.62) (11.9759, 58.62) (12.2848, 58.5225) (12.5178, 58.3572) (12.683, 58.1431) (12.786, 57.9128) (12.8348, 57.6744) (12.8348, 57.5742) knots 0 0 0 1 2 3 4 5 6 6 6
  line L70 (12.8348, 57.5742) -> (12.8348, 57.3276)
  point P0 (-54.8494, 0)
  constraints: 2 other
sketch "Esboço38" plane through (0, 0, -54.8494) normal (1, 0, 0) x (0, 0, -1)
  point P0 (-54.8494, 0)
extrude "Extrusão29" cut sketch "Esboço37" against normal blind 2
sketch "Esboço39" plane through (0, 0, -54.8494) normal (1, 0, 0) x (0, 0, -1)
  line L0 (-49.8494, 64) -> (-48.8494, 64)
  line L1 (15.1506, 64) -> (-49.8494, 64) projected
  line L2 (-48.8494, 64) -> (-48.8494, 63)
  line L3 (15.1506, 44) -> (12.1506, 44) projected
  line L4 (-48.8494, 63) -> (14.1506, 63)
  line L5 (14.1506, 63) -> (14.1506, 44)
  line L6 (14.1506, 44) -> (-48.8494, 44)
  line L7 (-48.8494, 44) -> (-48.8494, 63)
  line L8 (-46, 61) -> (-9, 61)
  line L9 (-9, 61) -> (-9, 58)
  line L10 (-9, 58) -> (-46, 58)
  line L11 (-46, 58) -> (-46, 61)
  line L12 (-46, 56) -> (-9, 56)
  line L13 (-9, 56) -> (-9, 53)
  line L14 (-9, 53) -> (-46, 53)
  line L15 (-46, 53) -> (-46, 56)
  line L16 (-46, 51) -> (-9, 51)
  line L17 (-9, 51) -> (-9, 48)
  line L18 (-9, 48) -> (-46, 48)
  line L19 (-46, 48) -> (-46, 51)
  point P0 (-54.8494, 0)
  dimension "d104" = 1
  dimension "d105" = 63
  constraints: 36 end point, 8 parallel, 4 horizontal, 4 perpendicular, 4 point on line, 1 vertical
  measures "d104" distance of L0.start L0.end
  measures "d105" distance of L5.end L6.end
extrude "Extrusão30" cut sketch "Esboço39" against normal blind 1
sketch "Esboço40" plane through (0, 58, -45.8494) normal (1, 0, 0) x (0, 0, -1)
  line L0 (0, 3) -> (-37, 3) projected
  line L1 (-37, 0) -> (0, 0) projected
  line L2 (-37, 3) -> (0, 3)
  line L3 (0, 3) -> (0, 0)
  line L4 (0, 0) -> (-37, 0)
  line L5 (-37, 0) -> (-37, 3)
  line L6 (0, -5) -> (0, -2) projected
  line L7 (-37, -2) -> (0, -2)
  line L8 (0, -2) -> (0, -5)
  line L9 (0, -5) -> (-37, -5)
  line L10 (-37, -5) -> (-37, -2)
  line L11 (0, -7) -> (-37, -7) projected
  line L12 (-37, -10) -> (0, -10) projected
  line L13 (-37, -7) -> (0, -7)
  line L14 (0, -7) -> (0, -10)
  line L15 (0, -10) -> (-37, -10)
  line L16 (-37, -10) -> (-37, -7)
  point P0 (-45.8494, -58)
  constraints: 24 end point, 6 parallel, 3 horizontal, 3 perpendicular, 1 point on line
extrude "Extrusão31" cut sketch "Esboço40" against normal through all
sketch "Esboço41" plane through (-65, 12, -31.5) normal (1, 0, 0) x (0, 0, -1)
  point P0 (-31.5, -12)
sketch "Esboço42" plane through (0, 44, 0) normal (0, 1, 0) x (1, 0, 0)
  line L0 (-55.5, 70) -> (-70, 70) projected
  line L1 (-70, 70) -> (-70, 65)
  line L2 (-70, 5) -> (-70, 70) projected
  line L3 (-70, 70) -> (-65, 70) construction
  line L4 (-70, 65) -> (-65, 65)
  line L5 (-65, 8) -> (-65, 67) projected
  line L6 (-70, 5) -> (-65, 5)
  line L7 (-65, 5) -> (-65, 10)
  line L8 (-65, 10) -> (-70, 10)
  line L9 (-70, 10) -> (-70, 5)
  line L10 (-10, 67) -> (-10, 8) projected
  line L11 (-5, 70) -> (-10, 70)
  line L12 (-10, 70) -> (-10, 65)
  line L13 (-10, 65) -> (-5, 65)
  line L14 (-5, 65) -> (-5, 70)
  line L15 (-5, 5) -> (-10, 5)
  line L16 (-10, 5) -> (-10, 10)
  line L17 (-10, 10) -> (-5, 10)
  line L18 (-5, 10) -> (-5, 5)
  circle A0 centre (-65, 65) radius 2.5
  circle A1 centre (-10, 65) radius 2.5
  circle A2 centre (-10, 10) radius 2.5
  circle A3 centre (-65, 10) radius 2.5
  point P0 (0, 0)
  dimension "d110" = 5
  dimension "d111" = 90
  dimension "d112" = 5
  dimension "d113" = 5
  dimension "d114" = 5
  dimension "d115" = 5
  dimension "d116" = 5
  constraints: 30 end point, 6 parallel, 5 perpendicular, 4 centre point, 4 coincident, 4 horizontal, 3 point on line, 1 collinear
  measures "d110" distance of L0.end L1.end
  measures "d111" angle of L1 L3
  measures "d112" distance of L1.end L4.end
  measures "d113" diameter of A0
  measures "d114" diameter of A1
  measures "d115" diameter of A2
  measures "d116" diameter of A3
extrude "Extrusão32" add sketch "Esboço42" against normal blind 44 contours A3 L5 L8 | L8 L5 L7 A3 | L7 L5 A3 | A0 L5 L4 | L4 L5 A0 | L12 A1 L13 L10 | L10 A1 L12 | L13 A1 L10 | A2 L17 L10 | L10 L16 A2 | L17 A2 L16 L10
sketch "Esboço43" plane through (0, 44, 0) normal (0, 1, 0) x (1, 0, 0)
  circle A0 centre (-10, 65) radius 1.5
  circle A1 centre (-10, 10) radius 1.5
  circle A2 centre (-65, 10) radius 1.5
  circle A3 centre (-65, 65) radius 1.5
  point P0 (0, 0)
  dimension "d119" = 3
  dimension "d120" = 3
  dimension "d121" = 3
  dimension "d122" = 3
  constraints: 4 centre point
  measures "d119" diameter of A0
  measures "d120" diameter of A1
  measures "d121" diameter of A2
  measures "d122" diameter of A3
extrude "Extrusão33" cut sketch "Esboço43" against normal blind 10
thread "Rosca5" size "M3x0.5" class "6H" standard "ANSI Metric M Profile" length 11
thread "Rosca6" size "M3x0.5" class "6H" standard "ANSI Metric M Profile" length 11
thread "Rosca7" size "M3x0.5" class "6H" standard "ANSI Metric M Profile" length 11
thread "Rosca8" size "M3x0.5" class "6H" standard "ANSI Metric M Profile" length 11
sketch "Esboço44" plane through (0, 64, 0) normal (0, 1, 0) x (1, 0, 0)
  line L0 (-5, 75) -> (-70, 75) projected
  line L1 (-5, 75) -> (-13, 75)
  line L2 (-13, 75) -> (-13, 72.5)
  line L3 (-5, 70) -> (-19.5, 70) projected
  line L4 (-70, 75) -> (-62, 75)
  line L5 (-62, 75) -> (-62, 72.5)
  arc A0 (-75, 5) -> (-70, 0) centre (-70, 5) ccw projected
  line L6 (-70, 0) -> (-62, 0)
  line L7 (-62, 0) -> (-62, 2.5)
  arc A1 (-5, 0) -> (0, 5) centre (-5, 5) ccw projected
  line L8 (-5, 0) -> (-13, 0)
  line L9 (-70, 0) -> (-5, 0) projected
  line L10 (-13, 0) -> (-13, 2.5)
  line L11 (-19.5, 5) -> (-5, 5) projected
  circle A2 centre (-62, 72.5) radius 1
  circle A3 centre (-13, 72.5) radius 1
  circle A4 centre (-13, 2.5) radius 1
  circle A5 centre (-62, 2.5) radius 1
  point P0 (0, 0)
  dimension "d133" = 8
  dimension "d134" = 2.5
  dimension "d135" = 8
  dimension "d136" = 2.5
  dimension "d137" = 2.5
  dimension "d138" = 8
  dimension "d139" = 2
  dimension "d140" = 2
  dimension "d141" = 2
  dimension "d142" = 2
  constraints: 16 end point, 4 centre point, 4 coincident, 4 perpendicular, 3 point on line, 1 horizontal, 1 tangent
  measures "d133" distance of L0.start L1.end
  measures "d134" distance of L1.end L2.end
  measures "d135" distance of L0.end L4.end
  measures "d136" distance of L4.end L5.end
  measures "d137" distance of L6.end L7.end
  measures "d138" distance of L8.start L8.end
  measures "d139" diameter of A2
  measures "d140" diameter of A3
  measures "d141" diameter of A4
  measures "d142" diameter of A5
extrude "Extrusão34" cut sketch "Esboço44" against normal blind 10
thread "Rosca9" size "M2x0.4" class "6H" standard "ANSI Metric M Profile" length 11
thread "Rosca10" size "M2x0.4" class "6H" standard "ANSI Metric M Profile" length 11
thread "Rosca11" size "M2x0.4" class "6H" standard "ANSI Metric M Profile" length 11
thread "Rosca12" size "M2x0.4" class "6H" standard "ANSI Metric M Profile" length 11
sketch "Esboço45" plane through (-75, 0, -20.1506) normal (-1, 0, 0) x (0, 0, 1)
  line L0 (15.1506, 64) -> (14.1506, 64)
  line L1 (14.1506, 64) -> (14.1506, 63)
  line L2 (-48.8494, 63) -> (-48.8494, 44) projected
  line L3 (14.1506, 63) -> (-48.8494, 63)
  line L4 (-48.8494, 63) -> (-48.8494, 44)
  line L5 (-48.8494, 44) -> (14.1506, 44)
  line L6 (14.1506, 44) -> (14.1506, 63)
  point P0 (20.1506, 0)
  dimension "d153" = 1
  constraints: 12 end point, 2 horizontal, 2 parallel, 2 perpendicular
  measures "d153" distance of L0.start L0.end
extrude "Extrusão35" cut sketch "Esboço45" against normal blind 1
sketch "Esboço46" plane through (-74, 0, -20.1506) normal (-1, 0, 0) x (0, 0, 1)
  line L0 (-48.8675, 66.6126) -> (-26.17, 66.6126) construction
  line L1 (-26.17, 66.6126) -> (-26.17, 47.407) construction
  line L2 (-26.17, 47.407) -> (-48.8675, 47.407) construction
  line L3 (-48.8675, 47.407) -> (-48.8675, 66.6126) construction
  spline S0 degree 2 poles (-43.9834, 57.2713) (-43.9834, 57.0789) (-44.0782, 56.7754) (-44.2435, 56.5397) (-44.4548, 56.3745) (-44.6878, 56.2688) (-44.9235, 56.22) (-44.9831, 56.22) knots 0 0 0 1 2 3 4 5 6 6 6
  line L4 (-44.9831, 56.22) -> (-43.8533, 55.2446)
  line L5 (-43.8533, 55.2446) -> (-44.7528, 55.2446)
  line L6 (-44.7528, 55.2446) -> (-45.8827, 56.22)
  line L7 (-45.8827, 56.22) -> (-46.2972, 56.22)
  line L8 (-46.2972, 56.22) -> (-46.2972, 56.8486)
  line L9 (-46.2972, 56.8486) -> (-45.0265, 56.8486)
  spline S1 degree 2 poles (-45.0265, 56.8486) (-44.9398, 56.8567) (-44.7826, 56.919) (-44.6743, 57.0247) (-44.6119, 57.1737) (-44.6119, 57.2713) knots 0 0 0 1 2 3 4 4 4
  line L10 (-44.6119, 57.2713) -> (-44.6119, 57.6127)
  spline S2 degree 2 poles (-44.6119, 57.6127) (-44.6119, 57.6479) (-44.6255, 57.675) (-44.6417, 57.6858) (-44.6716, 57.6885) (-44.6851, 57.6885) knots 0 0 0 1 2 3 4 4 4
  line L11 (-44.6851, 57.6885) -> (-46.4245, 57.6885)
  line L12 (-46.4245, 57.6885) -> (-46.4245, 55.2446)
  line L13 (-46.4245, 55.2446) -> (-47.0558, 55.2446)
  line L14 (-47.0558, 55.2446) -> (-47.0558, 58.0001)
  spline S3 degree 2 poles (-47.0558, 58.0001) (-47.0558, 58.0678) (-47.0098, 58.1816) (-46.9231, 58.2683) (-46.8066, 58.3171) (-46.7388, 58.3171) knots 0 0 0 1 2 3 4 4 4
  line L15 (-46.7388, 58.3171) -> (-44.6851, 58.3171)
  spline S4 degree 2 poles (-44.6851, 58.3171) (-44.4927, 58.3171) (-44.2218, 58.1762) (-44.0565, 57.9649) (-43.9834, 57.721) (-43.9834, 57.6154) knots 0 0 0 1 2 3 4 4 4
  line L16 (-43.9834, 57.6154) -> (-43.9834, 57.2713)
  spline S5 degree 2 poles (-40.9732, 56.0493) (-40.9732, 55.903) (-41.0491, 55.6673) (-41.1737, 55.4885) (-41.3363, 55.3611) (-41.5151, 55.2826) (-41.6993, 55.2446) (-41.7806, 55.2446) knots 0 0 0 1 2 3 4 5 6 6 6
  line L17 (-41.7806, 55.2446) -> (-42.756, 55.2446)
  spline S6 degree 2 poles (-42.756, 55.2446) (-42.8779, 55.2446) (-43.157, 55.3286) (-43.3981, 55.5183) (-43.558, 55.8272) (-43.558, 56.0493) knots 0 0 0 1 2 3 4 4 4
  line L18 (-43.558, 56.0493) -> (-43.558, 56.7809)
  spline S7 degree 2 poles (-43.558, 56.7809) (-43.558, 57.0003) (-43.3981, 57.3065) (-43.157, 57.4989) (-42.8752, 57.5828) (-42.756, 57.5828) knots 0 0 0 1 2 3 4 4 4
  line L19 (-42.756, 57.5828) -> (-41.7806, 57.5828)
  spline S8 degree 2 poles (-41.7806, 57.5828) (-41.5612, 57.5828) (-41.2496, 57.423) (-41.0599, 57.1819) (-40.9732, 56.9001) (-40.9732, 56.7809) knots 0 0 0 1 2 3 4 4 4
  line L20 (-40.9732, 56.7809) -> (-40.9732, 56.0493)
  spline S9 degree 2 poles (-41.6045, 56.7782) (-41.6045, 56.8703) (-41.6939, 56.9543) (-41.7806, 56.9543) knots 0 0 0 1 2 2 2
  line L21 (-41.7806, 56.9543) -> (-42.7533, 56.9543)
  spline S10 degree 2 poles (-42.7533, 56.9543) (-42.8427, 56.9543) (-42.9267, 56.8703) (-42.9267, 56.7809) knots 0 0 0 1 2 2 2
  line L22 (-42.9267, 56.7809) -> (-42.9267, 56.0493)
  spline S11 degree 2 poles (-42.9267, 56.0493) (-42.9267, 55.9599) (-42.8427, 55.8732) (-42.7533, 55.8732) knots 0 0 0 1 2 2 2
  line L23 (-42.7533, 55.8732) -> (-41.7806, 55.8732)
  spline S12 degree 2 poles (-41.7806, 55.8732) (-41.6885, 55.8732) (-41.6045, 55.9599) (-41.6045, 56.0493) knots 0 0 0 1 2 2 2
  line L24 (-41.6045, 56.0493) -> (-41.6045, 56.7782)
  spline S13 degree 2 poles (-37.9685, 56.0493) (-37.9685, 55.968) (-38.0064, 55.7865) (-38.085, 55.6104) (-38.2096, 55.4478) (-38.3912, 55.3205) (-38.6269, 55.2446) (-38.7732, 55.2446) knots 0 0 0 1 2 3 4 5 6 6 6
  line L25 (-38.7732, 55.2446) -> (-39.7486, 55.2446)
  spline S14 degree 2 poles (-39.7486, 55.2446) (-39.8326, 55.2446) (-40.0114, 55.2826) (-40.1902, 55.3611) (-40.3528, 55.4858) (-40.4774, 55.6646) (-40.5533, 55.9003) (-40.5533, 56.0493) knots 0 0 0 1 2 3 4 5 6 6 6
  line L26 (-40.5533, 56.0493) -> (-40.5533, 58.5338)
  line L27 (-40.5533, 58.5338) -> (-39.922, 58.5338)
  line L28 (-39.922, 58.5338) -> (-39.922, 56.0493)
  spline S15 degree 2 poles (-39.922, 56.0493) (-39.922, 55.9653) (-39.8244, 55.8732) (-39.7486, 55.8732) knots 0 0 0 1 2 2 2
  line L29 (-39.7486, 55.8732) -> (-38.7732, 55.8732)
  spline S16 degree 2 poles (-38.7732, 55.8732) (-38.6892, 55.8732) (-38.5998, 55.968) (-38.5998, 56.0493) knots 0 0 0 1 2 2 2
  line L30 (-38.5998, 56.0493) -> (-38.5998, 56.7809)
  spline S17 degree 2 poles (-38.5998, 56.7809) (-38.5998, 56.8621) (-38.6946, 56.9543) (-38.7732, 56.9543) knots 0 0 0 1 2 2 2
  line L31 (-38.7732, 56.9543) -> (-39.7919, 56.9543)
  line L32 (-39.7919, 56.9543) -> (-39.7919, 57.5828)
  line L33 (-39.7919, 57.5828) -> (-38.7732, 57.5828)
  spline S18 degree 2 poles (-38.7732, 57.5828) (-38.6946, 57.5828) (-38.5104, 57.5449) (-38.3316, 57.4636) (-38.169, 57.339) (-38.0444, 57.1602) (-37.9685, 56.9245) (-37.9685, 56.7809) knots 0 0 0 1 2 3 4 5 6 6 6
  line L34 (-37.9685, 56.7809) -> (-37.9685, 56.0493)
  spline S19 degree 2 poles (-34.9936, 56.0493) (-34.9936, 55.903) (-35.0694, 55.6673) (-35.1941, 55.4885) (-35.3566, 55.3611) (-35.5354, 55.2826) (-35.7197, 55.2446) (-35.801, 55.2446) knots 0 0 0 1 2 3 4 5 6 6 6
  line L35 (-35.801, 55.2446) -> (-36.7764, 55.2446)
  spline S20 degree 2 poles (-36.7764, 55.2446) (-36.8983, 55.2446) (-37.1773, 55.3286) (-37.4185, 55.5183) (-37.5783, 55.8272) (-37.5783, 56.0493) knots 0 0 0 1 2 3 4 4 4
  line L36 (-37.5783, 56.0493) -> (-37.5783, 56.7809)
  spline S21 degree 2 poles (-37.5783, 56.7809) (-37.5783, 57.0003) (-37.4185, 57.3065) (-37.1773, 57.4989) (-36.8956, 57.5828) (-36.7764, 57.5828) knots 0 0 0 1 2 3 4 4 4
  line L37 (-36.7764, 57.5828) -> (-35.801, 57.5828)
  spline S22 degree 2 poles (-35.801, 57.5828) (-35.5815, 57.5828) (-35.2699, 57.423) (-35.0803, 57.1819) (-34.9936, 56.9001) (-34.9936, 56.7809) knots 0 0 0 1 2 3 4 4 4
  line L38 (-34.9936, 56.7809) -> (-34.9936, 56.0493)
  spline S23 degree 2 poles (-35.6249, 56.7782) (-35.6249, 56.8703) (-35.7143, 56.9543) (-35.801, 56.9543) knots 0 0 0 1 2 2 2
  line L39 (-35.801, 56.9543) -> (-36.7736, 56.9543)
  spline S24 degree 2 poles (-36.7736, 56.9543) (-36.8631, 56.9543) (-36.947, 56.8703) (-36.947, 56.7809) knots 0 0 0 1 2 2 2
  line L40 (-36.947, 56.7809) -> (-36.947, 56.0493)
  spline S25 degree 2 poles (-36.947, 56.0493) (-36.947, 55.9599) (-36.8631, 55.8732) (-36.7736, 55.8732) knots 0 0 0 1 2 2 2
  line L41 (-36.7736, 55.8732) -> (-35.801, 55.8732)
  spline S26 degree 2 poles (-35.801, 55.8732) (-35.7089, 55.8732) (-35.6249, 55.9599) (-35.6249, 56.0493) knots 0 0 0 1 2 2 2
  line L42 (-35.6249, 56.0493) -> (-35.6249, 56.7782)
  line L43 (-35.549, 57.7861) -> (-36.2887, 58.16)
  line L44 (-36.2887, 58.16) -> (-37.0256, 57.7861)
  line L45 (-37.0256, 57.7861) -> (-37.3101, 58.1925)
  line L46 (-37.3101, 58.1925) -> (-36.2887, 58.775)
  line L47 (-36.2887, 58.775) -> (-35.2672, 58.1925)
  line L48 (-35.2672, 58.1925) -> (-35.549, 57.7861)
  line L49 (-31.4822, 55.2446) -> (-32.1108, 55.2446)
  line L50 (-32.1108, 55.2446) -> (-32.1108, 55.9789)
  line L51 (-32.1108, 55.9789) -> (-33.9261, 55.9789)
  line L52 (-33.9261, 55.9789) -> (-33.9261, 55.2446)
  line L53 (-33.9261, 55.2446) -> (-34.5574, 55.2446)
  line L54 (-34.5574, 55.2446) -> (-34.5574, 56.7809)
  spline S27 degree 2 poles (-34.5574, 56.7809) (-34.5574, 57.1168) (-34.3243, 57.6831) (-33.9125, 58.0895) (-33.3517, 58.3171) (-33.0211, 58.3171) knots 0 0 0 1 2 3 4 4 4
  line L55 (-33.0211, 58.3171) -> (-31.7992, 58.3171)
  spline S28 degree 2 poles (-31.7992, 58.3171) (-31.7342, 58.3171) (-31.6177, 58.2683) (-31.5282, 58.1816) (-31.4822, 58.0651) (-31.4822, 58.0001) knots 0 0 0 1 2 3 4 4 4
  line L56 (-31.4822, 58.0001) -> (-31.4822, 55.2446)
  line L57 (-33.9261, 56.6048) -> (-32.1108, 56.6048)
  line L58 (-32.1108, 56.6048) -> (-32.1108, 57.6885)
  line L59 (-32.1108, 57.6885) -> (-33.0211, 57.6885)
  spline S29 degree 2 poles (-33.0211, 57.6885) (-33.0428, 57.6885) (-33.1972, 57.675) (-33.3977, 57.6181) (-33.6199, 57.5043) (-33.8041, 57.3038) (-33.9261, 57.0003) (-33.9261, 56.7809) knots 0 0 0 1 2 3 4 5 6 6 6
  line L60 (-33.9261, 56.7809) -> (-33.9261, 56.6048)
  spline S30 degree 2 poles (-27.8001, 57.0247) (-27.8001, 56.8323) (-27.8949, 56.5289) (-28.0602, 56.2959) (-28.2715, 56.1306) (-28.5046, 56.0249) (-28.743, 55.9789) (-28.8459, 55.9789) knots 0 0 0 1 2 3 4 5 6 6 6
  line L61 (-28.8459, 55.9789) -> (-30.1139, 55.9789)
  line L62 (-30.1139, 55.9789) -> (-30.1139, 56.6048)
  line L63 (-30.1139, 56.6048) -> (-28.8432, 56.6048)
  spline S31 degree 2 poles (-28.8432, 56.6048) (-28.7538, 56.6129) (-28.5994, 56.6752) (-28.491, 56.7809) (-28.4287, 56.9299) (-28.4287, 57.0247) knots 0 0 0 1 2 3 4 4 4
  line L64 (-28.4287, 57.0247) -> (-28.4287, 57.2658)
  spline S32 degree 2 poles (-28.4287, 57.2658) (-28.4395, 57.3607) (-28.5018, 57.5178) (-28.6048, 57.6289) (-28.7484, 57.6885) (-28.8459, 57.6885) knots 0 0 0 1 2 3 4 4 4
  line L65 (-28.8459, 57.6885) -> (-30.0679, 57.6885)
  spline S33 degree 2 poles (-30.0679, 57.6885) (-30.1546, 57.6885) (-30.2413, 57.6018) (-30.2413, 57.5151) knots 0 0 0 1 2 2 2
  line L66 (-30.2413, 57.5151) -> (-30.2413, 55.2446)
  line L67 (-30.2413, 55.2446) -> (-30.8726, 55.2446)
  line L68 (-30.8726, 55.2446) -> (-30.8726, 57.5151)
  spline S34 degree 2 poles (-30.8726, 57.5151) (-30.8726, 57.7319) (-30.71, 58.0434) (-30.4716, 58.2331) (-30.1898, 58.3171) (-30.0706, 58.3171) knots 0 0 0 1 2 3 4 4 4
  line L69 (-30.0706, 58.3171) -> (-28.8459, 58.3171)
  spline S35 degree 2 poles (-28.8459, 58.3171) (-28.659, 58.3171) (-28.3501, 58.2196) (-28.1171, 58.0543) (-27.9518, 57.8402) (-27.8489, 57.6099) (-27.8001, 57.3715) (-27.8001, 57.2713) knots 0 0 0 1 2 3 4 5 6 6 6
  line L70 (-27.8001, 57.2713) -> (-27.8001, 57.0247)
  point P0 (20.1506, 0)
  constraints: 2 other
extrude "Extrusão36" cut sketch "Esboço46" against normal blind 1
sketch "Esboço47" plane through (-5, 44, -75) normal (0, 0, -1) x (-1, 0, 0)
  point P0 (-5, -44)
sketch "Esboço48" plane through (0, 44, 0) normal (0, 1, 0) x (1, 0, 0)
  point P0 (0, 0)
sketch "Esboço49" plane through (0, 44, 0) normal (0, 1, 0) x (1, 0, 0)
  line L0 (-65, 65) -> (-62.5, 65)
  arc A0 (-65, 62.5) -> (-63.5, 67) centre (-65, 65) ccw projected
  line L1 (-62.5, 65) -> (-62.5, 67.5)
  line L2 (-62.5, 65) -> (-62.5, 51.5)
  line L3 (-41, 51.5) -> (-65, 51.5) projected
  line L4 (-65, 51.5) -> (-62.5, 51.5)
  circle A1 centre (-65, 65) radius 1.5 projected
  line L5 (-65, 65) -> (-65, 67.5)
  line L6 (-65, 67.5) -> (-62.5, 67.5)
  line L7 (-62.5, 67.5) -> (-62.5, 51.5)
  line L8 (-62.5, 51.5) -> (-65, 51.5)
  line L9 (-65, 51.5) -> (-65, 67.5)
  arc A2 (-11.5, 67) -> (-10, 62.5) centre (-10, 65) ccw projected
  line L10 (-12.5, 65) -> (-12.5, 67.5)
  line L11 (-10, 62.5) -> (-10, 12.5) projected
  line L12 (-12.5, 67.5) -> (-10, 67.5)
  line L13 (-10, 67.5) -> (-10, 51.5)
  line L14 (-10, 51.5) -> (-12.5, 51.5)
  line L15 (-12.5, 51.5) -> (-12.5, 67.5)
  circle A3 centre (-10, 10) radius 1.5 projected
  line L16 (-10, 10) -> (-10, 7.5)
  line L17 (-10, 7.5) -> (-12.5, 7.5)
  line L18 (-12.5, 7.5) -> (-10, 7.5)
  line L19 (-10, 7.5) -> (-10, 23.5)
  line L20 (-10, 23.5) -> (-12.5, 23.5)
  line L21 (-12.5, 23.5) -> (-12.5, 7.5)
  line L22 (-65, 23.5) -> (-41, 23.5) projected
  line L23 (-65, 23.5) -> (-62.5, 23.5)
  line L24 (-62.5, 23.5) -> (-62.5, 7.5)
  line L25 (-62.5, 7.5) -> (-65, 7.5)
  line L26 (-65, 7.5) -> (-65, 23.5)
  arc A4 (-65, 7.5) -> (-65, 12.5) centre (-65, 10) ccw
  point P0 (0, 0)
  point P1 (-10, 62.5)
  point P2 (-65, 66.5)
  point P3 (-63.5, 65)
  point P4 (-10, 8.5)
  point P5 (-10, 11.5)
  point P6 (-62.5, 10)
  dimension "d171" = 2.5
  dimension "d172" = 2.5
  dimension "d173" = 16
  constraints: 48 end point, 8 parallel, 6 horizontal, 5 vertical, 4 perpendicular, 4 point on circle, 4 point on line, 2 tangent, 1 centre point, 1 collinear
  measures "d171" distance of L0.end L1.end
  measures "d172" distance of L16.start L16.end
  measures "d173" distance of L19.end L18.end
sketch "Esboço50" plane through (0, 44, 0) normal (0, 1, 0) x (1, 0, 0)
  point P0 (0, 0)
sketch "Esboço51" plane through (0, 44, 0) normal (0, 1, 0) x (1, 0, 0)
  point P0 (0, 0)
sketch "Esboço52" plane through (0, 44, 0) normal (0, 1, 0) x (1, 0, 0)
  point P0 (0, 0)